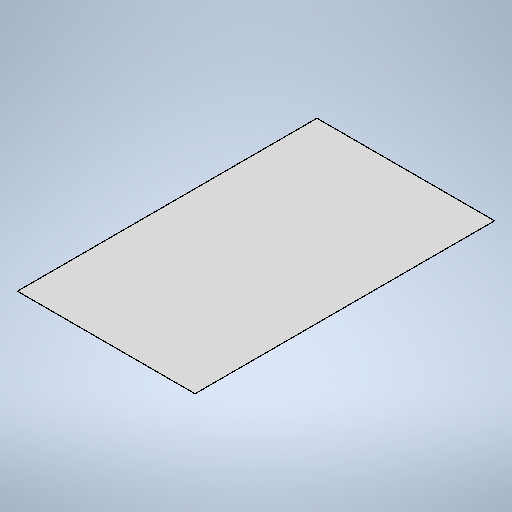
# Autodesk Inventor part: PNS-0116 floor sheet 6
Saved by Autodesk Inventor 2025.1 (Build 291241020, 241B)
## iProperties
Created: 2025-03-10
Part Number: PNS-0116 floor sheet 6
Material: Stainless Steel
Document SubType Name: Sheet Metal
Designer: user
Stock Number: PNS-0111 floor sheet 2
Mass: 72000 g
Surface Area: 90180 cm^2
Volume: 9000 cm^3
Density: 8 g/cm^3
Sheet Metal Rule: AISI304 2mm Die16
Sheet Metal Width: 1340.000 mm
Sheet Metal Length: 2260.000 mm
Sheet Metal Area: 3028400.000 mm^2
Appearance: Default
Flat Pattern Width: 134 cm
Flat Pattern Length: 226 cm
Flat Pattern Area: 30284 cm^2
Author: admin
Autodesk Inventor part; units mm, degrees
ref_plane "YZ Plane" through (0, 0, 0) normal (1, 0, 0) x (0, 1, 0)
ref_plane "XZ Plane" through (0, 0, 0) normal (0, 1, 0) x (-1, 0, 0)
ref_plane "XY Plane" through (0, 0, 0) normal (0, 0, 1) x (1, 0, 0)
sketch "Sketch1" plane through (0, 0, 0) normal (0, 0, 1) x (1, 0, 0)
  line L0 (-670, -1130) -> (670, -1130)
  line L1 (670, -1130) -> (670, 1130)
  line L2 (670, 1130) -> (-670, 1130)
  line L3 (-670, 1130) -> (-670, -1130)
  line L4 (-670, -1130) -> (670, 1130) construction
  line L5 (670, -1130) -> (-670, 1130) construction
  point P0 (0, 0)
  dimension "d154" = 1340
  dimension "d155" = 2260
  measures "d154" distance of L1.end L2.end
  measures "d155" distance of L0.end L1.end
extrude "Plate5" add sketch "Sketch1" along normal blind 2
body "Solid3"
